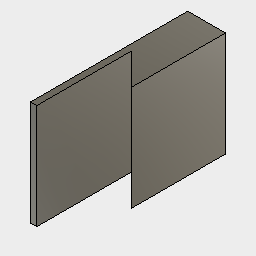
generic_holder (Autodesk Fusion 360 design; units mm, degrees)
Autodesk Fusion 360 part; units mm, degrees
sketch "Sketch1" plane through (0, 0, 0) normal (0, 0, 1) x (1, 0, 0) in component "generic_holder"
  line L0 (0, 0) -> (-15, 15)
  line L1 (-15, 15) -> (-15, 45)
  line L2 (-15, 45) -> (0, 45)
  line L3 (0, 45) -> (0, 0)
  line L4 (-15, 45) -> (-18, 45)
  line L5 (-18, 45) -> (-18, -30)
  line L6 (-18, -30) -> (-15, -30)
  line L7 (-15, -30) -> (-15, 45)
  dimension "d2" = 15
  dimension "d3" = 30
  dimension "d4" = 75
  dimension "d5" = 3
  dimension "d9" = 45
  measures "d2" distance of L1.end L2.end
  measures "d3" distance of L0.end L1.end
  measures "d4" distance of L1.end L6.end
  measures "d5" distance of L1.end L4.end
  measures "d9" distance of L2.end L0.start
extrude "Extrude1" add sketch "Sketch1" along normal blind 50 in component "generic_holder"
component "generic_holder" placed x (1, 0, 0) y (0, 1, 0) z (0, 0, 1) at (0, 0, 0)
equation "d2 = cleat_thickness"
equation "d3 = cleat_short_hight"
equation "d4 = front_plate_hight"
equation "d5 = cleat_front_plate_thickness"
equation "cleat_thickness = 15 mm" comment "Cleat thickness"
equation "cleat_long_hight = 45 mm" comment "Cleat long side hight"
equation "cleat_short_hight = 30 mm" comment "Cleat short side hight"
equation "d9 = cleat_long_hight"
equation "cleat_front_plate_thickness = 3 mm" comment "Front plate thickness"
equation "front_plate_hight = 75 mm" comment "Front plate ight"
equation "cleat_width = 50 mm" comment "Cleat width"
equation "d13 = cleat_width"
named bodies: "holder"
